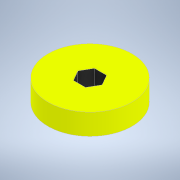
# Autodesk Inventor part: 2 in Compliance Wheel
Saved by Autodesk Inventor 2021 (Build 250183000, 183)
## iProperties
Created: 2021-01-16
Part Number: 2 in Compliance Wheel
Material: Rubber, Silicone
Document SubType Name: Modeling
Designer: magda
Density: 1.25 g/cm^3
Appearance: Rubber - Black
Author: magda
Autodesk Inventor part; units mm, degrees
ref_plane "YZ Plane" through (0, 0, 0) normal (1, 0, 0) x (0, 1, 0)
ref_plane "XZ Plane" through (0, 0, 0) normal (0, 1, 0) x (-1, 0, 0)
ref_plane "XY Plane" through (0, 0, 0) normal (0, 0, 1) x (1, 0, 0)
sketch "Sketch1" plane through (0, 0, 0) normal (0, 1, 0) x (-1, 0, 0)
  circle A0 centre (0, 0) radius 25.4
  line L0 (3.6662, -6.35) -> (-3.6662, -6.35)
  line L1 (-3.6662, -6.35) -> (-7.3323, 0)
  line L2 (-7.3323, 0) -> (-3.6662, 6.35)
  line L3 (-3.6662, 6.35) -> (3.6662, 6.35)
  line L4 (3.6662, 6.35) -> (7.3323, 0)
  line L5 (7.3323, 0) -> (3.6662, -6.35)
  dimension "d0" = 50.8
  dimension "d4" = 12.7
  dimension "d5" = 6.35
  constraints: 12 end point, 1 centre point, 1 coincident, 1 horizontal, 13 other
  measures "d0" diameter of A0
  measures "d4" distance between parallel lines of L3 L0
  measures "d5" distance from line of A0.centre L0
extrude "Extrusion1" add sketch "Sketch1" along normal blind 12.7
body "Solid1"
